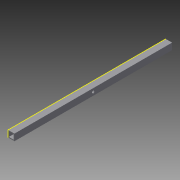
# Autodesk Inventor part: 5x5mm Box Aluminum
Saved by Autodesk Inventor 2013 (Build 170138000, 138)
## iProperties
Created: 2013-10-02
Part Number: 5x5mm Box Aluminum
Material: Aluminum 6061
Document SubType Name: Modeling
Designer: cobrooks
Density: 1 g/cm^3
Author: cobrooks
Autodesk Inventor part; units mm, degrees
ref_plane "YZ Plane" through (0, 0, 0) normal (1, 0, 0) x (0, 1, 0)
ref_plane "XZ Plane" through (0, 0, 0) normal (0, 1, 0) x (-1, 0, 0)
ref_plane "XY Plane" through (0, 0, 0) normal (0, 0, 1) x (1, 0, 0)
sketch "Sketch1" plane through (0, 0, 0) normal (0, 0, 1) x (1, 0, 0)
  line L0 (-6.35, -6.35) -> (6.35, -6.35)
  line L1 (6.35, -6.35) -> (6.35, 6.35)
  line L2 (6.35, 6.35) -> (-6.35, 6.35)
  line L3 (-6.35, 6.35) -> (-6.35, -6.35)
  line L4 (-6.35, -6.35) -> (6.35, 6.35) construction
  line L5 (6.35, -6.35) -> (-6.35, 6.35) construction
  line L6 (-4.572, -4.572) -> (4.572, -4.572)
  line L7 (4.572, -4.572) -> (4.572, 4.572)
  line L8 (4.572, 4.572) -> (-4.572, 4.572)
  line L9 (-4.572, 4.572) -> (-4.572, -4.572)
  line L10 (-4.572, -4.572) -> (4.572, 4.572) construction
  line L11 (4.572, -4.572) -> (-4.572, 4.572) construction
  point P0 (0, 0)
  dimension "d0" = 12.7
  dimension "d1" = 12.7
  dimension "d5" = 1.778
  constraints: 24 end point, 4 midpoint, 4 parallel, 2 horizontal, 2 perpendicular, 1 point on line
  measures "d0" distance of L2.end L1.end
  measures "d1" distance between parallel lines of L0 L2
  measures "d5" distance between parallel lines of L1 L7
extrude "Extrusion1" add sketch "Sketch1" along normal blind 304.8
sketch "Sketch3" plane through (6.35, 6.35, 304.8) normal (1, 0, 0) x (0, 0, -1)
  point P0 (304.8, -6.35)
  point P1 (152.4, -6.35)
hole "Hole1" at (6.35, 0, 152.4) direction (-1, 0, 0) diameter 4.7625 depth 25.4 tip angle 118
sketch "Sketch4" plane through (-6.35, -6.35, 0) normal (-1, 0, 0) x (0, 0, 1)
  line L0 (0, 12.7) -> (0, 0) projected
  line L1 (304.8, 12.7) -> (304.8, 0) projected
  circle A0 centre (298.45, 6.35) radius 2.1336
  circle A1 centre (6.35, 6.35) radius 2.1336
  point P0 (0, 6.35)
  dimension "d13" = 4.2672
  dimension "d14" = 6.35
  dimension "d15" = 4.2672
  dimension "d16" = 6.35
  constraints: 2 centre point
  measures "d13" diameter of A0
  measures "d14" distance from line of L1 A0.centre
  measures "d15" diameter of A1
  measures "d16" distance from line of L0 A1.centre
extrude "Extrusion2" cut sketch "Sketch4" against normal blind 12.7
body "Solid1"
